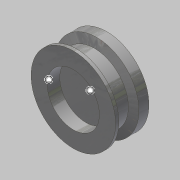
# Autodesk Inventor part: CHECK VALVE DUALPLATE WAFER 316L DN100
Saved by Autodesk Inventor 2017 (Build 210142000, 142)
## iProperties
Created: 2015-03-19
Part Number: CHECK VALVE DUALPLATE WAFER 316L DN100
Material: 316L
Document SubType Name: Modeling
Designer: m_crauwels
Density: 8 g/cm^3
Appearance: Steel
Mass: 365.342 g
Surface Area: 480.363 cm^2
Volume: 45.6678 cm^3
Description: BV40-PN10/PN16
Catalog Web Link: http://www.pocketbrewery.com
PipeDiameter: 100.000 mm
DiamExt: 162.000 mm
Thickness: 64.000 mm
Author: m_crauwels
Autodesk Inventor part; units mm, degrees
ref_plane "YZ Plane" through (0, 0, 0) normal (1, 0, 0) x (0, 1, 0)
ref_plane "XZ Plane" through (0, 0, 0) normal (0, 1, 0) x (-1, 0, 0)
ref_plane "XY Plane" through (0, 0, 0) normal (0, 0, 1) x (1, 0, 0)
sketch "Sketch1" plane through (0, 0, 0) normal (0, 1, 0) x (-1, 0, 0)
  line L0 (32, 0) -> (-32, 0) construction
  line L1 (32, 81) -> (-32, 81)
  line L2 (-32, 81) -> (-32, 50)
  line L3 (32, 50) -> (-32, 50)
  line L4 (32, 50) -> (32, 81)
  line L5 (8, 0) -> (-8, 0)
  line L6 (-8, 0) -> (-8, 50)
  line L7 (-8, 50) -> (8, 50)
  line L8 (8, 50) -> (8, 0)
  line L9 (8, 0) -> (-8, 50) construction
  line L10 (-8, 0) -> (8, 50) construction
  point P0 (0, 25)
  point P1 (0, 50)
  point P2 (0, 0)
  point P3 (0, 0)
  dimension "Thickness" = 64
  dimension "DiamExt" = 162
  dimension "PipeDiameter" = 100
  dimension "d8" = 16
  constraints: 22 end point, 6 midpoint, 4 perpendicular, 2 horizontal, 2 parallel, 1 coincident, 1 point on line
  measures "Thickness" distance of L1.start L1.end
  measures "DiamExt" diameter of L1 L0
  measures "PipeDiameter" diameter of L3 L0
  measures "d8" distance of L6.end L7.end
revolve "Revolution1" add sketch "Sketch1" angle 360 about axis through (-32, 0, 0) along (1, 0, 0)
sketch "Sketch6" plane through (0, 0, 0) normal (0, 1, 0) x (-1, 0, 0)
  line L0 (-32, 81) -> (32, 81) projected
  line L1 (32, 50) -> (8, 50) projected
  line L2 (25.6, 81) -> (21.3128, 65)
  line L3 (21.3128, 65) -> (-8.5128, 65)
  line L4 (-8.5128, 65) -> (-12.8, 81)
  line L5 (32, -81) -> (32, 81) projected
  line L6 (44.8, 0) -> (-44.8, 0) projected
  point P0 (0, 0)
  dimension "d26" = 15
  dimension "d27" = 75
  dimension "d28" = 44.8
  dimension "d29" = 6.4
  constraints: 6 end point, 2 point on line, 1 equal length, 1 horizontal
  measures "d26" distance between parallel lines of L3 L1
  measures "d27" angle of L0 L2
  measures "d28" distance from line of L4.end L5
  measures "d29" distance of L2.start L0.end
revolve "Revolution2" cut sketch "Sketch6" angle 360 about axis through (-10, 0, 0) along (1, 0, 0)
equation "\"d8\" = 0.25 * Thickness"
equation "\"d28\" = 0.7 * Thickness"
equation "\"d29\" = 0.1 * Thickness"
body "Solid1"
